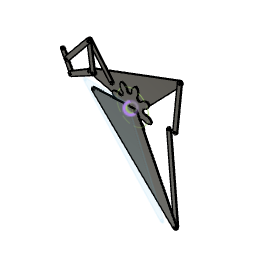
CAD (Autodesk Fusion 360 design; units mm, degrees)
description: Spur Gear; Module: 2.0; Num Teeth: 8; Pressure Angle: 20.0; Backlash: 0.00 mm
Autodesk Fusion 360 part; units mm, degrees
note: some values were not read from the file. Set by a fixed rule: which sketch regions a step uses.
(part 1 of 2)
sketch "Sketch2" plane through (0, 0, 0) normal (0, 1, 0) x (1, 0, 0)
  line L0 (20.2187, -3.6863) -> (18.4977, -4.9158)
  arc A0 (18.4977, -4.9158) -> (19.6603, -6.5431) centre (19.079, -5.7294) ccw
  line L1 (19.6603, -6.5431) -> (21.3813, -5.3137)
  arc A1 (21.3813, -5.3137) -> (20.2187, -3.6863) centre (20.8, -4.5) ccw
  line L2 (20.8, -4.5) -> (19.079, -5.7294) construction
  line L3 (19.079, -5.7294) -> (20.8, -4.5)
  circle A2 centre (19.079, -5.7294) radius 0.5
  circle A3 centre (20.8, -4.5) radius 0.5
  dimension "d10" = 2
  dimension "d11" = 1
  dimension "d12" = 1
  constraint tangent L0 A0
  constraint tangent A0 L1
  constraint parallel L0 L1
  constraint tangent L1 A1
  constraint tangent L0 A1
  constraint coincident A0.centre L2.end
  constraint coincident A1.centre L2.start
  constraint concentric A0 A2
  constraint concentric A1 A3
  measures "d10" diameter of A0
  measures "d11" diameter of A2
  measures "d12" diameter of A3
sketch "Sketch3" plane through (0, 0, 0) normal (0, 1, 0) x (1, 0, 0)
  line L0 (40.363, -4.4753) -> (54.2331, 34.1031)
  arc A0 (54.2331, 34.1031) -> (52.351, 34.7797) centre (53.2921, 34.4414) ccw
  line L1 (52.351, 34.7797) -> (38.481, -3.7987)
  arc A1 (38.481, -3.7987) -> (40.363, -4.4753) centre (39.422, -4.137) ccw
  line L2 (39.422, -4.137) -> (53.2921, 34.4414) construction
  line L3 (39.422, -4.137) -> (53.2921, 34.4414)
  circle A2 centre (39.422, -4.137) radius 0.5
  circle A3 centre (53.2921, 34.4414) radius 0.5
  dimension "d17" = 2
  dimension "d18" = 1
  dimension "d19" = 1
  constraint tangent L0 A0
  constraint tangent A0 L1
  constraint parallel L0 L1
  constraint tangent L1 A1
  constraint tangent L0 A1
  constraint coincident A1.centre L2.start
  constraint coincident A0.centre L2.end
  constraint concentric A1 A2
  constraint concentric A0 A3
  measures "d17" diameter of A0
  measures "d18" diameter of A2
  measures "d19" diameter of A3
extrude "Extrude2" add sketch "Sketch3" against normal blind 0.5 makes body 1
sketch "Sketch4" plane through (0, 0, 0) normal (0, 1, 0) x (1, 0, 0)
  line L0 (41.629, -4.9251) -> (52.2449, -24.6941)
  arc A0 (52.2449, -24.6941) -> (54.0069, -23.7479) centre (53.1259, -24.221) ccw
  line L1 (54.0069, -23.7479) -> (43.391, -3.9789)
  arc A1 (43.391, -3.9789) -> (41.629, -4.9251) centre (42.51, -4.452) ccw
  line L2 (42.51, -4.452) -> (53.1259, -24.221) construction
  line L3 (42.51, -4.452) -> (53.1259, -24.221)
  circle A2 centre (42.51, -4.452) radius 0.5
  circle A3 centre (53.1259, -24.221) radius 0.5
  dimension "d24" = 2
  dimension "d25" = 1
  dimension "d26" = 1
  constraint tangent L0 A0
  constraint tangent A0 L1
  constraint parallel L0 L1
  constraint tangent L1 A1
  constraint tangent L0 A1
  constraint coincident A1.centre L2.start
  constraint coincident A0.centre L2.end
  constraint concentric A1 A2
  constraint concentric A0 A3
  measures "d24" diameter of A0
  measures "d25" diameter of A2
  measures "d26" diameter of A3
extrude "Extrude3" add sketch "Sketch4" against normal blind 0.5 separate body makes body 2
sketch "Sketch5" plane through (0, 0, 0) normal (0, 1, 0) x (1, 0, 0)
  line L0 (-13.1989, -13.1062) -> (-9.6831, -4.2011)
  arc A0 (-9.6831, -4.2011) -> (-11.5434, -3.4667) centre (-10.6133, -3.8339) ccw
  line L1 (-11.5434, -3.4667) -> (-15.0591, -12.3718)
  arc A1 (-15.0591, -12.3718) -> (-13.1989, -13.1062) centre (-14.129, -12.739) ccw
  line L2 (-14.129, -12.739) -> (-10.6133, -3.8339) construction
  line L3 (-14.129, -12.739) -> (-10.6133, -3.8339)
  circle A2 centre (-14.129, -12.739) radius 0.5
  circle A3 centre (-10.6133, -3.8339) radius 0.5
  dimension "d32" = 2
  dimension "d33" = 1
  dimension "d34" = 1
  constraint tangent L0 A0
  constraint tangent A0 L1
  constraint parallel L0 L1
  constraint tangent L1 A1
  constraint tangent L0 A1
  constraint coincident A1.centre L2.start
  constraint coincident A0.centre L2.end
  constraint concentric A1 A2
  constraint concentric A0 A3
  measures "d32" diameter of A0
  measures "d33" diameter of A2
  measures "d34" diameter of A3
extrude "Extrude4" add sketch "Sketch5" against normal blind 0.5 separate body makes body 3
copy_body "Body->Comp1" bodies 2 removing the originals makes body 4 in component "Component"
copy_body "Body->Comp2" bodies 1 removing the originals makes body 5 in component "Component'"
copy_body "Body->Comp4" bodies 3 removing the originals makes body 6 in component "Component''"
sketch "Sketch8" plane through (0, 0, 0) normal (0, 1, 0) x (1, 0, 0)
  line L0 (-5, -5) -> (5, -5)
  line L1 (5, -5) -> (5, 2.5)
  line L2 (5, 2.5) -> (-5, 2.5)
  line L3 (-5, 2.5) -> (-5, -5)
  constraint horizontal L0
  constraint vertical L1
  constraint horizontal L2
  constraint vertical L3
extrude "Extrude5" add sketch "Sketch8" along normal blind 0.5 separate body makes body 7
copy_body "Body->Comp5" bodies 7 removing the originals makes body 8 in component "Component'''"
sketch "Sketch9" plane through (0, 0, 0) normal (0, 1, 0) x (1, 0, 0)
  line L0 (-1, -1) -> (1, -1)
  line L1 (1, -1) -> (1, 1)
  line L2 (1, 1) -> (-1, 1)
  line L3 (-1, 1) -> (-1, -1)
  constraint horizontal L0
  constraint vertical L1
  constraint horizontal L2
  constraint vertical L3
extrude "Extrude6" add sketch "Sketch9" along normal blind 0.5 separate body makes body 9
copy_body "Body->Comp6" bodies 9 removing the originals makes body 10 in component "Component''''"
sketch "Sketch10" plane through (0, 0, 0) normal (0, 1, 0) x (1, 0, 0)
  line L0 (-1, -1) -> (1, -1)
  line L1 (1, -1) -> (1, 1)
  line L2 (1, 1) -> (-1, 1)
  line L3 (-1, 1) -> (-1, -1)
  constraint horizontal L0
  constraint vertical L1
  constraint horizontal L2
  constraint vertical L3
extrude "Extrude7" add sketch "Sketch10" along normal blind 0.5 separate body makes body 11
copy_body "Body->Comp7" bodies 11 removing the originals makes body 12 in component "Component'''''"
sketch "Sketch11" plane through (0, 0, 0) normal (0, 1, 0) x (1, 0, 0)
  line L0 (-0.5, -0.5) -> (0.5, -0.5)
  line L1 (0.5, -0.5) -> (0.5, 0.5)
  line L2 (0.5, 0.5) -> (-0.5, 0.5)
  line L3 (-0.5, 0.5) -> (-0.5, -0.5)
  constraint horizontal L0
  constraint vertical L1
  constraint horizontal L2
  constraint vertical L3
extrude "Extrude8" add sketch "Sketch11" along normal blind 0.5 separate body makes body 13
copy_body "Body->Comp8" bodies 13 removing the originals makes body 14 in component "Component''''''"
sketch "Sketch14" plane through (0, 0, 0) normal (0, 1, 0) x (1, 0, 0)
  line L0 (0, 0) -> (4.9713, -9.3835)
  line L1 (4.9713, -9.3835) -> (6.8938, -11.5466)
  line L2 (6.8938, -11.5466) -> (0, 0)
  line L3 (-19.2227, 34.1473) -> (4.144, -9.9579)
  line L4 (4.144, -9.9579) -> (13.1804, -20.1253)
  line L5 (13.1804, -20.1253) -> (-19.2227, 34.1473)
  circle A0 centre (0, 0) radius 1
  circle A1 centre (6.8938, -11.5466) radius 1
  circle A2 centre (4.9713, -9.3835) radius 1
  circle A3 centre (6.8938, -11.5466) radius 0.5
  circle A4 centre (4.9713, -9.3835) radius 0.5
  circle A5 centre (0, 0) radius 0.5
  dimension "d87" = 10.619
  dimension "d88" = 2.894
  dimension "d89" = 13.448
  dimension "d90" = 1
  dimension "d91" = 1
  dimension "d92" = 1
  dimension "d93" = 1
  constraint coincident L0.start L2.end
  constraint coincident L1.end L2.start
  constraint tangent L4 A1
  constraint coincident L0.end L1.start
  constraint tangent L3 A2
  constraint concentric A1 A3
  constraint concentric A2 A4
  measures "d87" distance of L0.start L0.end
  measures "d88" distance of L0.end L1.end
  measures "d89" distance of L1.end L0.start
  measures "d91" diameter of A3
  measures "d92" diameter of A4
  measures "d93" diameter of A5
extrude "Extrude10" add sketch "Sketch14" against normal blind 0.5 separate body contours L0 L2 A0 A5 | L0 L2 A0 A5 | L0 L2 A0 A2 | L0 L3 A0 A2 | L2 L5 A0 A1 A2 | L0 L1 L2 A2 A4 | L0 L1 A2 A4 | L2 A2 | L1 L2 A1 A2 | L1 L4 A1 A2 | L1 L2 A1 A3 | L1 L2 A1 A3 makes body 15
copy_body "Body->Comp9" bodies 15 removing the originals makes body 16 in component "Component'''''''"
sketch "Sketch15" plane through (0, 0, 0) normal (0, 1, 0) x (1, 0, 0)
  line L0 (-1, 0) -> (-1, -13.5)
  arc A0 (-1, -13.5) -> (1, -13.5) centre (0, -13.5) ccw
  line L1 (1, -13.5) -> (1, 0)
  arc A1 (1, 0) -> (-1, 0) centre (0, 0) ccw
  line L2 (0, 0) -> (0, -13.5) construction
  circle A2 centre (0, -13.5) radius 0.5
  circle A3 centre (0, 0) radius 0.5
  dimension "d100" = 2
  dimension "d101" = 1
  dimension "d102" = 1
  constraint tangent L0 A0
  constraint tangent A0 L1
  constraint parallel L0 L1
  constraint tangent L1 A1
  constraint tangent L0 A1
  constraint vertical L2
  constraint coincident A1.centre L2.start
  constraint concentric A0 A2
  constraint concentric A1 A3
  measures "d100" diameter of A0
  measures "d101" diameter of A2
  measures "d102" diameter of A3
extrude "Extrude11" add sketch "Sketch15" against normal blind 0.5 separate body makes body 17
copy_body "Body->Comp10" bodies 17 removing the originals makes body 18 in component "Component''''''''"
sketch "Sketch16" plane through (0, 0, 0) normal (0, 1, 0) x (1, 0, 0)
  line L0 (-2, -2) -> (2, -2)
  line L1 (2, -2) -> (2, 30)
  line L2 (2, 30) -> (-2, 30)
  line L3 (-2, 30) -> (-2, -2)
  constraint horizontal L0
  constraint vertical L1
  constraint horizontal L2
  constraint vertical L3
extrude "Extrude12" add sketch "Sketch16" along normal blind 0.5 separate body makes body 19
copy_body "Body->Comp11" bodies 19 removing the originals makes body 20 in component "Component'''''''''"
sketch "Sketch17" plane through (0, 0, 0) normal (0, 1, 0) x (1, 0, 0)
  line L0 (5.9221, 49.648) -> (29.8072, 28.8562)
  line L1 (5.9221, 49.648) -> (-16.9692, 41.844)
  line L2 (-16.9692, 41.844) -> (29.8072, 28.8562)
  line L3 (6.1444, 50.7803) -> (33.7942, 26.7114)
  line L4 (-20.355, 41.7463) -> (33.7942, 26.7114)
  line L5 (6.1444, 50.7803) -> (-20.355, 41.7463)
  circle A0 centre (29.8072, 28.8562) radius 1
  circle A1 centre (-16.9692, 41.844) radius 1
  circle A2 centre (5.9221, 49.648) radius 1
  circle A3 centre (5.9221, 49.648) radius 0.5
  circle A4 centre (29.8072, 28.8562) radius 0.5
  circle A5 centre (-16.9692, 41.844) radius 0.5
  dimension "d111" = 50
  dimension "d112" = 31.667
  dimension "d113" = 24.185
  dimension "d114" = 48.546
  dimension "d115" = 1
  dimension "d116" = 1
  dimension "d117" = 1
  dimension "d118" = 1
  constraint coincident L0.end L2.end
  constraint tangent L4 A0
  constraint coincident L1.end L2.start
  constraint tangent L4 A1
  constraint coincident L0.start L1.start
  constraint tangent L3 A2
  constraint concentric A2 A3
  constraint concentric A0 A4
  constraint concentric A1 A5
  measures "d111" distance of origin L0.start
  measures "d112" distance of L0.start L0.end
  measures "d113" distance of L0.start L1.end
  measures "d114" distance of L1.end L0.end
  measures "d116" diameter of A3
  measures "d117" diameter of A4
  measures "d118" diameter of A5
extrude "Extrude13" add sketch "Sketch17" against normal blind 0.5 separate body contours L0 L1 A2 A3 | L0 L1 A2 A3 | L0 L3 A0 A2 | L0 L1 L2 A0 A1 A2 | L1 L5 A1 A2 | L0 L2 A0 A4 | L0 L2 A0 A4 | L1 L2 A1 A5 | L1 L2 A1 A5 | L2 L4 A0 A1 makes body 21
copy_body "Body->Comp12" bodies 21 removing the originals makes body 22 in component "Component''''''''''"
sketch "Sketch18" plane through (0, 0, 0) normal (0, 1, 0) x (1, 0, 0)
  line L0 (0, 40) -> (28.0014, 75.7058)
  line L1 (0, 40) -> (-20.2217, 44.9555)
  line L2 (-20.2217, 44.9555) -> (28.0014, 75.7058)
  line L3 (0.3887, 38.8752) -> (32.4039, 79.6992)
  line L4 (-22.7316, 44.541) -> (32.4039, 79.6992)
  line L5 (0.3887, 38.8752) -> (-22.7316, 44.541)
  circle A0 centre (0, 40) radius 1
  circle A1 centre (-20.2217, 44.9555) radius 1
  circle A2 centre (28.0014, 75.7058) radius 1
  circle A3 centre (-20.2217, 44.9555) radius 0.5
  circle A4 centre (0, 40) radius 0.5
  circle A5 centre (28.0014, 75.7058) radius 0.5
  dimension "d129" = 40
  dimension "d130" = 45.376
  dimension "d131" = 20.82
  dimension "d132" = 57.193
  dimension "d133" = 1
  dimension "d134" = 1
  dimension "d135" = 1
  dimension "d136" = 1
  constraint coincident L0.end L2.end
  constraint coincident L0.start L1.start
  constraint tangent L5 A0
  constraint coincident L1.end L2.start
  constraint tangent L5 A1
  constraint tangent L3 A2
  constraint concentric A1 A3
  constraint concentric A0 A4
  constraint concentric A2 A5
  measures "d129" distance of origin L0.start
  measures "d130" distance of L0.start L0.end
  measures "d131" distance of L0.start L1.end
  measures "d132" distance of L1.end L0.end
  measures "d134" diameter of A3
  measures "d135" diameter of A4
  measures "d136" diameter of A5
extrude "Extrude14" add sketch "Sketch18" against normal blind 0.5 separate body contours L0 L1 A0 A4 | L0 L1 A0 A4 | L0 L1 L2 A0 A1 A2 | L0 L3 A0 A2 | L1 L5 A0 A1 | L0 L2 A2 A5 | L0 L2 A2 A5 | L1 L2 A1 A3 | L1 L2 A1 A3 | L2 L4 A1 A2 makes body 23
copy_body "Body->Comp13" bodies 23 removing the originals makes body 24 in component "Component'''''''''''"
sketch "Sketch19" plane through (0, 0, 0) normal (0, 1, 0) x (1, 0, 0)
  circle A0 centre (0, 20) radius 1
  circle A1 centre (0, 20) radius 0.5
  dimension "d151" = 20
  dimension "d152" = 2
  dimension "d153" = 1
  constraint concentric A0 A1
  measures "d151" distance of origin A0.centre
  measures "d152" diameter of A0
  measures "d153" diameter of A1
extrude "Extrude15" add sketch "Sketch19" along normal blind 0.5 separate body makes body 25
chamfer "Chamfer1" distance 0.1 angle 45 1 edges at (-0.9323, 0, -19.6384) on bodies 25
chamfer "Chamfer2" distance 0.1 angle 45 1 edges at (-0.9323, 0.5, -19.6384) on bodies 25
chamfer "Chamfer3" distance 0.1 angle 45 2 edges at (-0.4662, 0, -20.1808) (-0.4662, 0.5, -20.1808) on bodies 25
copy_body "Body->Comp14" bodies 25 removing the originals makes body 26 in component "Component''''''''''''"
move_face "OffsetFaces1" offset -16 1 faces at (-0.6667, 0.1667, 2) on bodies 20 in component "Component'''''''''"
sketch "Sketch20" plane through (0, 0, 0) normal (0, 1, 0) x (1, 0, 0)
  line L0 (-10, 0) -> (-14, 0)
  line L1 (-14, 0) -> (-14, 16)
  line L2 (-10, 0) -> (-10, 16)
  line L3 (-10, 16) -> (-14, 16)
  dimension "d168" = 10
  dimension "d169" = 4
  dimension "d170" = 16
  dimension "d171" = 16
  constraint perpendicular L0 L1
  constraint perpendicular L1 L3
  measures "d168" distance of origin L0.start
  measures "d169" distance of L0.start L0.end
  measures "d170" distance of L0.end L1.end
  measures "d171" distance of L0.start L2.end
extrude "Extrude16" add sketch "Sketch20" along normal blind 0.5 separate body makes body 27
copy_body "Body->Comp15" bodies 27 removing the originals makes body 28 in component "Component'''''''''''''"
sketch "Sketch21" plane through (0, 0, 0) normal (0, 1, 0) x (1, 0, 0)
  line L0 (-39, 0) -> (-39, 17)
  arc A0 (-39, 17) -> (-41, 17) centre (-40, 17) ccw
  line L1 (-41, 17) -> (-41, 0)
  arc A1 (-41, 0) -> (-39, 0) centre (-40, 0) ccw
  line L2 (-40, 0) -> (-40, 17) construction
  circle A2 centre (-40, 0) radius 0.5
  circle A3 centre (-40, 17) radius 0.5
  dimension "d182" = 40
  dimension "d183" = 2
  dimension "d184" = 1
  dimension "d185" = 1
  constraint tangent L0 A0
  constraint tangent A0 L1
  constraint parallel L0 L1
  constraint tangent L1 A1
  constraint tangent L0 A1
  constraint concentric A1 A2
  constraint concentric A0 A3
  measures "d182" distance of origin A1.centre
  measures "d183" diameter of A0
  measures "d184" diameter of A2
  measures "d185" diameter of A3
extrude "Extrude17" add sketch "Sketch21" along normal blind 0.5 separate body makes body 29
copy_body "Body->Comp16" bodies 29 removing the originals makes body 30 in component "Component''''''''''''''"
sketch "Sketch22" plane through (0, 0, 0) normal (0, 1, 0) x (1, 0, 0)
  line L0 (-24, 0) -> (-24, 17)
  arc A0 (-24, 17) -> (-26, 17) centre (-25, 17) ccw
  line L1 (-26, 17) -> (-26, 0)
  arc A1 (-26, 0) -> (-24, 0) centre (-25, 0) ccw
  line L2 (-25, 0) -> (-25, 17) construction
  circle A2 centre (-25, 0) radius 0.5
  circle A3 centre (-25, 17) radius 0.5
  dimension "d189" = 25
  dimension "d190" = 2
  dimension "d191" = 1
  dimension "d192" = 1
  constraint tangent L0 A0
  constraint tangent A0 L1
  constraint parallel L0 L1
  constraint tangent L1 A1
  constraint tangent L0 A1
  constraint concentric A1 A2
  constraint concentric A0 A3
  measures "d189" distance of origin A1.centre
  measures "d190" diameter of A0
  measures "d191" diameter of A2
  measures "d192" diameter of A3
extrude "Extrude18" add sketch "Sketch22" along normal blind 0.5 separate body makes body 31
copy_body "Body->Comp17" bodies 31 removing the originals makes body 32 in component "Component'''''''''''''''"
sketch "Sketch23" plane through (0, 0, 0) normal (0, 1, 0) x (1, 0, 0)
  line L0 (-20, 0) -> (-16, 0)
  line L1 (-20, 0) -> (-20, 16)
  line L2 (-16, 0) -> (-16, 16)
  line L3 (-20, 16) -> (-16, 16)
  line L4 (-14.5, 0) -> (-10.5, 0)
  line L5 (-14.5, 0) -> (-14.5, 16)
  line L6 (-10.5, 0) -> (-10.5, 16)
  line L7 (-14.5, 16) -> (-10.5, 16)
  line L8 (-20, 17) -> (-16, 17)
  line L9 (-16, 17) -> (-16, 33)
  line L10 (-20, 17) -> (-20, 33)
  line L11 (-20, 33) -> (-16, 33)
  line L12 (-10, 17) -> (-14, 17)
  line L13 (-14, 17) -> (-14, 33)
  line L14 (-10, 17) -> (-10, 33)
  line L15 (-14, 33) -> (-10, 33)
  dimension "d195" = 4
  dimension "d196" = 16
  dimension "d197" = 16
  dimension "d198" = 4
  dimension "d199" = 16
  dimension "d200" = 16
  dimension "d201" = 16
  dimension "d202" = 16
  dimension "d203" = 4
  dimension "d204" = 16
  dimension "d205" = 16
  constraint perpendicular L0 L1
  constraint perpendicular L0 L2
  constraint perpendicular L4 L5
  constraint perpendicular L4 L6
  constraint horizontal L8
  constraint perpendicular L8 L9
  constraint perpendicular L8 L10
  constraint perpendicular L9 L12
  constraint perpendicular L12 L13
  constraint perpendicular L12 L14
  measures "d195" distance of L0.start L0.end
  measures "d196" distance of L0.start L1.end
  measures "d197" distance of L0.end L2.end
  measures "d198" distance of L4.start L4.end
  measures "d199" distance of L4.start L5.end
  measures "d200" distance of L4.end L6.end
  measures "d201" distance of L8.end L9.end
  measures "d202" distance of L8.start L10.end
  measures "d203" distance of L12.start L12.end
  measures "d204" distance of L12.end L13.end
  measures "d205" distance of L12.start L14.end
extrude "Extrude19" add sketch "Sketch23" along normal blind 0.5 separate body makes body 33 at (-11.8333, 0, -5.3333) makes body 34 at (-18.6667, 0, -22.3333) makes body 35 at (-18.6667, 0, -10.6667) makes body 36 at (-11.3333, 0, -22.3333)
copy_body "Body->Comp18" bodies 35 removing the originals makes body 37 in component "Component''''''''''''''''"
copy_body "Body->Comp19" bodies 33 removing the originals makes body 38 in component "Component'''''''''''''''''"
copy_body "Body->Comp20" bodies 34 removing the originals makes body 39 in component "Component''''''''''''''''''"
copy_body "Body->Comp21" bodies 36 removing the originals makes body 40 in component "Component'''''''''''''''''''"
sketch "Sketch24" plane through (0, 0, 0) normal (0, 1, 0) x (1, 0, 0)
  line L0 (0, 0) -> (0, -14.2)
  line L1 (0, -14.2) -> (3.4641, -12.2)
  line L2 (0, -14.2) -> (4, -14.2) construction
  line L3 (0, -14.2) -> (-3.4641, -12.2)
  dimension "d216" = 14.2
  dimension "d217" = 30
  dimension "d218" = 4
  constraint coincident L0.start origin
  constraint vertical L0
  constraint horizontal L2
  constraint symmetric L1.start L0 L2.start
  constraint symmetric L0 L1.end L3.end
  measures "d216" distance of L0.start L0.end
  measures "d217" angle of L1 L2
  measures "d218" distance of L0.end L1.end
sketch "Sketch1" plane through (0, 0, 0) normal (0, 0, 1) x (1, 0, 0) in component "Spur Gear (8 teeth)"
  circle A0 centre (0, 0) radius 5.5492
  circle A1 centre (0, 0) radius 0.5
extrude "Extrude1" add sketch "Sketch1" along normal blind 0.5 separate body makes body 41 in component "Spur Gear (8 teeth)"
sketch "Sketch2 (2)" plane through (0, 0, 0) normal (0, 0, 1) x (1, 0, 0) in component "Spur Gear (8 teeth)"
  spline S0 degree 5 poles (7.3504, -1.5763) (7.3577, -1.5779) (7.3723, -1.5807) (7.3943, -1.5841) (7.4239, -1.5871) (7.4612, -1.5888) (7.4987, -1.5889) (7.5364, -1.588) (7.5741, -1.5866) (7.6119, -1.5849) (7.6498, -1.5827) (7.6877, -1.5801) (7.7257, -1.5767) (7.7638, -1.5726) (7.802, -1.5677) (7.8402, -1.562) (7.8785, -1.5558) (7.9168, -1.549) (7.9551, -1.5418) (7.9935, -1.5341) (8.0319, -1.526) (8.0703, -1.5174) (8.1087, -1.5082) (8.1471, -1.4986) (8.1856, -1.4885) (8.224, -1.4779) (8.2624, -1.4668) (8.3009, -1.4553) (8.3393, -1.4434) (8.3778, -1.4311) (8.4162, -1.4183) (8.4546, -1.4051) (8.4929, -1.3915) (8.5313, -1.3774) (8.5696, -1.363) (8.608, -1.3481) (8.6462, -1.3328) (8.6845, -1.3172) (8.7227, -1.3011) (8.7609, -1.2847) (8.799, -1.2679) (8.8371, -1.2506) (8.8752, -1.2331) (8.9132, -1.2151) (8.9512, -1.1967) (8.9891, -1.178) (9.0269, -1.1589) (9.0647, -1.1395) (9.1025, -1.1197) (9.1401, -1.0995) (9.1778, -1.079) (9.2153, -1.0581) (9.2528, -1.0368) (9.2902, -1.0152) (9.3276, -0.9933) (9.3648, -0.971) (9.402, -0.9484) (9.4392, -0.9254) (9.4762, -0.9021) (9.5132, -0.8784) (9.55, -0.8544) (9.5868, -0.8301) (9.6235, -0.8055) (9.6602, -0.7805) (9.6967, -0.7552) (9.7331, -0.7295) (9.7695, -0.7036) (9.8057, -0.6773) (9.8418, -0.6507) (9.8779, -0.6238) (9.9138, -0.5965) (9.9425, -0.5745) (9.9639, -0.5578) (9.9782, -0.5466) (9.9854, -0.541) knots 0 0 0 0 0 0 0.01428571 0.02857143 0.04285714 0.05714286 0.07142857 0.08571429 0.1 0.11428571 0.12857143 0.14285714 0.15714286 0.17142857 0.18571429 0.2 0.21428571 0.22857143 0.24285714 0.25714286 0.27142857 0.28571429 0.3 0.31428571 0.32857143 0.34285714 0.35714286 0.37142857 0.38571429 0.4 0.41428571 0.42857143 0.44285714 0.45714286 0.47142857 0.48571429 0.5 0.51428571 0.52857143 0.54285714 0.55714286 0.57142857 0.58571429 0.6 0.61428571 0.62857143 0.64285714 0.65714286 0.67142857 0.68571429 0.7 0.71428571 0.72857143 0.74285714 0.75714286 0.77142857 0.78571429 0.8 0.81428571 0.82857143 0.84285714 0.85714286 0.87142857 0.88571429 0.9 0.91428571 0.92857143 0.94285714 0.95714286 0.97142857 0.98571429 1 1 1 1 1 1
  spline S1 degree 5 poles (7.3504, 1.5763) (7.3577, 1.5779) (7.3723, 1.5807) (7.3943, 1.5841) (7.4239, 1.5871) (7.4612, 1.5888) (7.4987, 1.5889) (7.5364, 1.588) (7.5741, 1.5866) (7.6119, 1.5849) (7.6498, 1.5827) (7.6877, 1.5801) (7.7257, 1.5767) (7.7638, 1.5726) (7.802, 1.5677) (7.8402, 1.562) (7.8785, 1.5558) (7.9168, 1.549) (7.9551, 1.5418) (7.9935, 1.5341) (8.0319, 1.526) (8.0703, 1.5174) (8.1087, 1.5082) (8.1471, 1.4986) (8.1856, 1.4885) (8.224, 1.4779) (8.2624, 1.4668) (8.3009, 1.4553) (8.3393, 1.4434) (8.3778, 1.4311) (8.4162, 1.4183) (8.4546, 1.4051) (8.4929, 1.3915) (8.5313, 1.3774) (8.5696, 1.363) (8.608, 1.3481) (8.6462, 1.3328) (8.6845, 1.3172) (8.7227, 1.3011) (8.7609, 1.2847) (8.799, 1.2679) (8.8371, 1.2506) (8.8752, 1.2331) (8.9132, 1.2151) (8.9512, 1.1967) (8.9891, 1.178) (9.0269, 1.1589) (9.0647, 1.1395) (9.1025, 1.1197) (9.1401, 1.0995) (9.1778, 1.079) (9.2153, 1.0581) (9.2528, 1.0368) (9.2902, 1.0152) (9.3276, 0.9933) (9.3648, 0.971) (9.402, 0.9484) (9.4392, 0.9254) (9.4762, 0.9021) (9.5132, 0.8784) (9.55, 0.8544) (9.5868, 0.8301) (9.6235, 0.8055) (9.6602, 0.7805) (9.6967, 0.7552) (9.7331, 0.7295) (9.7695, 0.7036) (9.8057, 0.6773) (9.8418, 0.6507) (9.8779, 0.6238) (9.9138, 0.5965) (9.9425, 0.5745) (9.9639, 0.5578) (9.9782, 0.5466) (9.9854, 0.541) knots 0 0 0 0 0 0 0.01428571 0.02857143 0.04285714 0.05714286 0.07142857 0.08571429 0.1 0.11428571 0.12857143 0.14285714 0.15714286 0.17142857 0.18571429 0.2 0.21428571 0.22857143 0.24285714 0.25714286 0.27142857 0.28571429 0.3 0.31428571 0.32857143 0.34285714 0.35714286 0.37142857 0.38571429 0.4 0.41428571 0.42857143 0.44285714 0.45714286 0.47142857 0.48571429 0.5 0.51428571 0.52857143 0.54285714 0.55714286 0.57142857 0.58571429 0.6 0.61428571 0.62857143 0.64285714 0.65714286 0.67142857 0.68571429 0.7 0.71428571 0.72857143 0.74285714 0.75714286 0.77142857 0.78571429 0.8 0.81428571 0.82857143 0.84285714 0.85714286 0.87142857 0.88571429 0.9 0.91428571 0.92857143 0.94285714 0.95714286 0.97142857 0.98571429 1 1 1 1 1 1
  arc A0 (9.9854, -0.541) -> (9.9854, 0.541) centre (0, 0) ccw
  line L0 (5.4161, -1.1636) -> (7.3504, -1.5763)
  line L1 (5.4161, 1.1636) -> (7.3504, 1.5763)
  line L2 (5.4161, -1.1636) -> (5.4161, 1.1636)
  point P0 (7.5292, -1.5881)
  point P1 (7.7124, -1.5778)
  point P2 (7.8984, -1.5522)
  point P3 (8.0864, -1.5135)
  point P4 (8.2759, -1.4628)
  point P5 (8.4663, -1.4008)
  point P6 (8.6575, -1.3282)
  point P7 (8.8489, -1.2451)
  point P8 (9.0403, -1.152)
  point P9 (9.2313, -1.049)
  point P10 (9.4216, -0.9362)
  point P11 (9.611, -0.8139)
  point P12 (9.799, -0.6821)
  point P13 (7.5292, 1.5881)
  point P14 (7.7124, 1.5778)
  point P15 (7.8984, 1.5522)
  point P16 (8.0864, 1.5135)
  point P17 (8.2759, 1.4628)
  point P18 (8.4663, 1.4008)
  point P19 (8.6575, 1.3282)
  point P20 (8.8489, 1.2451)
  point P21 (9.0403, 1.152)
  point P22 (9.2313, 1.049)
  point P23 (9.4216, 0.9362)
  point P24 (9.611, 0.8139)
  point P25 (9.799, 0.6821)
extrude "Extrude2'" add sketch "Sketch2 (2)" along normal blind 0.5 bodies 41 in component "Spur Gear (8 teeth)"
fillet "Fillet1" radius 1 2 edges at (5.4254, -1.1656, 0.25) (5.4254, 1.1656, 0.25) on bodies 41 in component "Spur Gear (8 teeth)"
pattern_circular "C-Pattern1" count 8 over 360 about axis through (0, 0, 0) along (0, 0, 1) of "Extrude2'", "Fillet1" in component "Spur Gear (8 teeth)"
sketch "Sketch3 (2)" plane through (0, 0, 0) normal (0, 0, 1) x (1, 0, 0) in component "Spur Gear (8 teeth)"
  circle A0 centre (0, 0) radius 8 construction
sketch "Sketch26" plane through (0, -1, 0) normal (0, -1, 0) x (1, 0, 0)
  circle A0 centre (36.5077, -36.7553) radius 0.5
  circle A1 centre (-2.0699, 5.468) radius 0.5
  circle A2 centre (18.7448, 4.9995) radius 0.5
  arc A3 (19.665, 5.391) -> (18.7673, 5.9992) centre (18.7448, 4.9995) ccw
  line L0 (18.7673, 5.9992) -> (-2.0474, 6.4678)
  arc A4 (-2.0474, 6.4678) -> (-2.8081, 4.7935) centre (-2.0699, 5.468) ccw
  line L1 (-2.8081, 4.7935) -> (35.7694, -37.4298)
  arc A5 (35.7694, -37.4298) -> (37.4279, -36.3638) centre (36.5077, -36.7553) ccw
  line L2 (37.4279, -36.3638) -> (19.665, 5.391)
  point P0 (20.8, 4.5)
sketch "Sketch27" plane through (0, -0.25, 0) normal (0, -1, 0) x (1, 0, 0)
  arc A0 (56.2039, -3.3739) -> (56.3228, -3.0869) centre (51.1385, -1.1076) ccw
  arc A1 (57.4657, -2.4656) -> (56.3228, -3.0869) centre (57.257, -3.4436) ccw
  line L0 (57.4657, -2.4656) -> (58.489, -2.684)
  spline S0 degree 5 poles (58.489, -2.684) (58.4963, -2.6855) (58.5109, -2.6883) (58.5329, -2.6918) (58.5625, -2.6948) (58.5998, -2.6964) (58.6373, -2.6965) (58.6749, -2.6956) (58.7127, -2.6943) (58.7505, -2.6925) (58.7883, -2.6904) (58.8263, -2.6877) (58.8643, -2.6844) (58.9024, -2.6802) (58.9405, -2.6753) (58.9788, -2.6697) (59.017, -2.6634) (59.0554, -2.6566) (59.0937, -2.6494) (59.1321, -2.6417) (59.1704, -2.6336) (59.2088, -2.625) (59.2472, -2.6159) (59.2857, -2.6063) (59.3241, -2.5961) (59.3625, -2.5855) (59.401, -2.5745) (59.4394, -2.563) (59.4779, -2.551) (59.5163, -2.5387) (59.5547, -2.5259) (59.5931, -2.5127) (59.6315, -2.4991) (59.6699, -2.4851) (59.7082, -2.4706) (59.7465, -2.4558) (59.7848, -2.4405) (59.823, -2.4248) (59.8613, -2.4088) (59.8994, -2.3923) (59.9376, -2.3755) (59.9757, -2.3583) (60.0137, -2.3407) (60.0517, -2.3227) (60.0897, -2.3044) (60.1276, -2.2857) (60.1655, -2.2666) (60.2033, -2.2471) (60.241, -2.2273) (60.2787, -2.2071) (60.3163, -2.1866) (60.3539, -2.1657) (60.3914, -2.1445) (60.4288, -2.1229) (60.4661, -2.1009) (60.5034, -2.0786) (60.5406, -2.056) (60.5777, -2.033) (60.6148, -2.0097) (60.6517, -1.9861) (60.6886, -1.9621) (60.7254, -1.9378) (60.7621, -1.9131) (60.7987, -1.8881) (60.8352, -1.8628) (60.8717, -1.8372) (60.908, -1.8112) (60.9442, -1.7849) (60.9804, -1.7583) (61.0164, -1.7314) (61.0524, -1.7041) (61.081, -1.6821) (61.1025, -1.6654) (61.1168, -1.6542) (61.1239, -1.6486) knots 0 0 0 0 0 0 0.01428571 0.02857143 0.04285714 0.05714286 0.07142857 0.08571429 0.1 0.11428571 0.12857143 0.14285714 0.15714286 0.17142857 0.18571429 0.2 0.21428571 0.22857143 0.24285714 0.25714286 0.27142857 0.28571429 0.3 0.31428571 0.32857143 0.34285714 0.35714286 0.37142857 0.38571429 0.4 0.41428571 0.42857143 0.44285714 0.45714286 0.47142857 0.48571429 0.5 0.51428571 0.52857143 0.54285714 0.55714286 0.57142857 0.58571429 0.6 0.61428571 0.62857143 0.64285714 0.65714286 0.67142857 0.68571429 0.7 0.71428571 0.72857143 0.74285714 0.75714286 0.77142857 0.78571429 0.8 0.81428571 0.82857143 0.84285714 0.85714286 0.87142857 0.88571429 0.9 0.91428571 0.92857143 0.94285714 0.95714286 0.97142857 0.98571429 1 1 1 1 1 1
  arc A2 (61.1239, -1.6486) -> (61.1239, -0.5666) centre (51.1385, -1.1076) ccw
  spline S1 degree 5 poles (61.1239, -0.5666) (61.1168, -0.561) (61.1025, -0.5499) (61.081, -0.5332) (61.0524, -0.5111) (61.0164, -0.4839) (60.9804, -0.457) (60.9442, -0.4304) (60.908, -0.4041) (60.8717, -0.3781) (60.8352, -0.3525) (60.7987, -0.3272) (60.7621, -0.3022) (60.7254, -0.2775) (60.6886, -0.2532) (60.6517, -0.2292) (60.6148, -0.2055) (60.5777, -0.1822) (60.5406, -0.1593) (60.5034, -0.1366) (60.4661, -0.1143) (60.4288, -0.0924) (60.3914, -0.0708) (60.3539, -0.0496) (60.3163, -0.0287) (60.2787, -0.0081) (60.241, 0.012) (60.2033, 0.0318) (60.1655, 0.0513) (60.1276, 0.0704) (60.0897, 0.0891) (60.0517, 0.1075) (60.0137, 0.1254) (59.9757, 0.143) (59.9376, 0.1602) (59.8994, 0.1771) (59.8613, 0.1935) (59.823, 0.2095) (59.7848, 0.2252) (59.7465, 0.2405) (59.7082, 0.2553) (59.6699, 0.2698) (59.6315, 0.2838) (59.5931, 0.2975) (59.5547, 0.3106) (59.5163, 0.3234) (59.4779, 0.3358) (59.4394, 0.3477) (59.401, 0.3592) (59.3625, 0.3703) (59.3241, 0.3809) (59.2857, 0.391) (59.2472, 0.4006) (59.2088, 0.4097) (59.1704, 0.4183) (59.1321, 0.4265) (59.0937, 0.4341) (59.0554, 0.4414) (59.017, 0.4481) (58.9788, 0.4544) (58.9405, 0.46) (58.9024, 0.4649) (58.8643, 0.4691) (58.8263, 0.4724) (58.7883, 0.4751) (58.7505, 0.4772) (58.7127, 0.479) (58.6749, 0.4804) (58.6373, 0.4812) (58.5998, 0.4811) (58.5625, 0.4795) (58.5329, 0.4765) (58.5109, 0.4731) (58.4963, 0.4702) (58.489, 0.4687) knots -1 -1 -1 -1 -1 -1 -0.98571429 -0.97142857 -0.95714286 -0.94285714 -0.92857143 -0.91428571 -0.9 -0.88571429 -0.87142857 -0.85714286 -0.84285714 -0.82857143 -0.81428571 -0.8 -0.78571429 -0.77142857 -0.75714286 -0.74285714 -0.72857143 -0.71428571 -0.7 -0.68571429 -0.67142857 -0.65714286 -0.64285714 -0.62857143 -0.61428571 -0.6 -0.58571429 -0.57142857 -0.55714286 -0.54285714 -0.52857143 -0.51428571 -0.5 -0.48571429 -0.47142857 -0.45714286 -0.44285714 -0.42857143 -0.41428571 -0.4 -0.38571429 -0.37142857 -0.35714286 -0.34285714 -0.32857143 -0.31428571 -0.3 -0.28571429 -0.27142857 -0.25714286 -0.24285714 -0.22857143 -0.21428571 -0.2 -0.18571429 -0.17142857 -0.15714286 -0.14285714 -0.12857143 -0.11428571 -0.1 -0.08571429 -0.07142857 -0.05714286 -0.04285714 -0.02857143 -0.01428571 0 0 0 0 0 0
  line L1 (58.489, 0.4687) -> (57.4657, 0.2503)
  arc A3 (56.3228, 0.8717) -> (57.4657, 0.2503) centre (57.257, 1.2283) ccw
  arc A4 (56.3228, 0.8717) -> (56.2039, 1.1586) centre (51.1385, -1.1076) ccw
  arc A5 (56.5727, 2.4061) -> (56.2039, 1.1586) centre (57.1167, 1.567) ccw
  line L2 (56.5727, 2.4061) -> (57.4507, 2.9753)
  spline S2 degree 5 poles (57.4507, 2.9753) (57.457, 2.9793) (57.4693, 2.9876) (57.4873, 3.0008) (57.5103, 3.0196) (57.5378, 3.0448) (57.5644, 3.0713) (57.5905, 3.0985) (57.6162, 3.1262) (57.6417, 3.1541) (57.6669, 3.1824) (57.6919, 3.2111) (57.7164, 3.2404) (57.7404, 3.2702) (57.7639, 3.3007) (57.7869, 3.3317) (57.8096, 3.3632) (57.8319, 3.3951) (57.8539, 3.4273) (57.8756, 3.4599) (57.897, 3.4927) (57.918, 3.526) (57.9387, 3.5596) (57.9591, 3.5936) (57.9791, 3.6279) (57.9988, 3.6626) (58.0182, 3.6976) (58.0372, 3.7329) (58.056, 3.7685) (58.0744, 3.8044) (58.0926, 3.8406) (58.1104, 3.8771) (58.1279, 3.9139) (58.1451, 3.9509) (58.162, 3.9882) (58.1786, 4.0258) (58.1948, 4.0637) (58.2108, 4.1018) (58.2265, 4.1402) (58.2418, 4.1788) (58.2569, 4.2177) (58.2717, 4.2568) (58.2862, 4.2962) (58.3003, 4.3357) (58.3142, 4.3756) (58.3278, 4.4156) (58.341, 4.4559) (58.354, 4.4964) (58.3667, 4.5371) (58.3791, 4.578) (58.3911, 4.6191) (58.4029, 4.6604) (58.4144, 4.7019) (58.4256, 4.7437) (58.4365, 4.7856) (58.4471, 4.8277) (58.4574, 4.87) (58.4674, 4.9125) (58.4771, 4.9552) (58.4865, 4.998) (58.4956, 5.0411) (58.5045, 5.0843) (58.513, 5.1277) (58.5212, 5.1712) (58.5291, 5.215) (58.5368, 5.2589) (58.5441, 5.3029) (58.5511, 5.3471) (58.5579, 5.3915) (58.5643, 5.436) (58.5705, 5.4807) (58.5751, 5.5166) (58.5785, 5.5435) (58.5807, 5.5615) (58.5818, 5.5705) knots 0 0 0 0 0 0 0.01428571 0.02857143 0.04285714 0.05714286 0.07142857 0.08571429 0.1 0.11428571 0.12857143 0.14285714 0.15714286 0.17142857 0.18571429 0.2 0.21428571 0.22857143 0.24285714 0.25714286 0.27142857 0.28571429 0.3 0.31428571 0.32857143 0.34285714 0.35714286 0.37142857 0.38571429 0.4 0.41428571 0.42857143 0.44285714 0.45714286 0.47142857 0.48571429 0.5 0.51428571 0.52857143 0.54285714 0.55714286 0.57142857 0.58571429 0.6 0.61428571 0.62857143 0.64285714 0.65714286 0.67142857 0.68571429 0.7 0.71428571 0.72857143 0.74285714 0.75714286 0.77142857 0.78571429 0.8 0.81428571 0.82857143 0.84285714 0.85714286 0.87142857 0.88571429 0.9 0.91428571 0.92857143 0.94285714 0.95714286 0.97142857 0.98571429 1 1 1 1 1 1
  arc A6 (58.5818, 5.5705) -> (57.8167, 6.3356) centre (51.1385, -1.1076) ccw
  spline S3 degree 5 poles (57.8167, 6.3356) (57.8077, 6.3345) (57.7897, 6.3323) (57.7627, 6.329) (57.7269, 6.3243) (57.6822, 6.3181) (57.6377, 6.3117) (57.5933, 6.3049) (57.5491, 6.2979) (57.505, 6.2906) (57.4612, 6.2829) (57.4174, 6.275) (57.3739, 6.2668) (57.3305, 6.2583) (57.2873, 6.2494) (57.2442, 6.2403) (57.2014, 6.2309) (57.1587, 6.2212) (57.1162, 6.2112) (57.0739, 6.2009) (57.0318, 6.1903) (56.9898, 6.1794) (56.9481, 6.1682) (56.9066, 6.1567) (56.8653, 6.145) (56.8241, 6.1329) (56.7832, 6.1205) (56.7425, 6.1078) (56.7021, 6.0949) (56.6618, 6.0816) (56.6217, 6.068) (56.5819, 6.0541) (56.5424, 6.04) (56.503, 6.0255) (56.4639, 6.0107) (56.425, 5.9957) (56.3864, 5.9803) (56.348, 5.9646) (56.3099, 5.9486) (56.272, 5.9324) (56.2344, 5.9158) (56.1971, 5.8989) (56.16, 5.8817) (56.1233, 5.8642) (56.0868, 5.8464) (56.0506, 5.8282) (56.0147, 5.8098) (55.9791, 5.7911) (55.9438, 5.772) (55.9088, 5.7526) (55.8741, 5.733) (55.8397, 5.7129) (55.8058, 5.6926) (55.7722, 5.6718) (55.7389, 5.6508) (55.706, 5.6294) (55.6735, 5.6077) (55.6413, 5.5857) (55.6094, 5.5634) (55.5779, 5.5408) (55.5469, 5.5177) (55.5164, 5.4942) (55.4866, 5.4702) (55.4573, 5.4457) (55.4286, 5.4208) (55.4003, 5.3955) (55.3723, 5.37) (55.3447, 5.3443) (55.3174, 5.3182) (55.291, 5.2917) (55.2658, 5.2642) (55.247, 5.2411) (55.2338, 5.2231) (55.2255, 5.2108) (55.2214, 5.2045) knots -1 -1 -1 -1 -1 -1 -0.98571429 -0.97142857 -0.95714286 -0.94285714 -0.92857143 -0.91428571 -0.9 -0.88571429 -0.87142857 -0.85714286 -0.84285714 -0.82857143 -0.81428571 -0.8 -0.78571429 -0.77142857 -0.75714286 -0.74285714 -0.72857143 -0.71428571 -0.7 -0.68571429 -0.67142857 -0.65714286 -0.64285714 -0.62857143 -0.61428571 -0.6 -0.58571429 -0.57142857 -0.55714286 -0.54285714 -0.52857143 -0.51428571 -0.5 -0.48571429 -0.47142857 -0.45714286 -0.44285714 -0.42857143 -0.41428571 -0.4 -0.38571429 -0.37142857 -0.35714286 -0.34285714 -0.32857143 -0.31428571 -0.3 -0.28571429 -0.27142857 -0.25714286 -0.24285714 -0.22857143 -0.21428571 -0.2 -0.18571429 -0.17142857 -0.15714286 -0.14285714 -0.12857143 -0.11428571 -0.1 -0.08571429 -0.07142857 -0.05714286 -0.04285714 -0.02857143 -0.01428571 0 0 0 0 0 0
  line L3 (55.2214, 5.2045) -> (54.6523, 4.3265)
  arc A7 (53.4048, 3.9577) -> (54.6523, 4.3265) centre (53.8132, 4.8705) ccw
  arc A8 (53.4048, 3.9577) -> (53.1178, 4.0766) centre (51.1385, -1.1076) ccw
  arc A9 (52.4965, 5.2195) -> (53.1178, 4.0766) centre (53.4745, 5.0108) ccw
  line L4 (52.4965, 5.2195) -> (52.7149, 6.2428)
  spline S4 degree 5 poles (52.7149, 6.2428) (52.7164, 6.2501) (52.7193, 6.2647) (52.7227, 6.2867) (52.7257, 6.3163) (52.7273, 6.3536) (52.7274, 6.3911) (52.7266, 6.4287) (52.7252, 6.4665) (52.7234, 6.5043) (52.7213, 6.5422) (52.7186, 6.5801) (52.7153, 6.6181) (52.7111, 6.6562) (52.7062, 6.6944) (52.7006, 6.7326) (52.6943, 6.7709) (52.6875, 6.8092) (52.6803, 6.8475) (52.6726, 6.8859) (52.6645, 6.9242) (52.6559, 6.9626) (52.6468, 7.0011) (52.6372, 7.0395) (52.6271, 7.0779) (52.6165, 7.1164) (52.6054, 7.1548) (52.5939, 7.1933) (52.582, 7.2317) (52.5696, 7.2701) (52.5568, 7.3085) (52.5436, 7.3469) (52.53, 7.3853) (52.516, 7.4237) (52.5015, 7.462) (52.4867, 7.5003) (52.4714, 7.5386) (52.4557, 7.5769) (52.4397, 7.6151) (52.4232, 7.6533) (52.4064, 7.6914) (52.3892, 7.7295) (52.3716, 7.7675) (52.3536, 7.8056) (52.3353, 7.8435) (52.3166, 7.8814) (52.2975, 7.9193) (52.278, 7.9571) (52.2582, 7.9948) (52.238, 8.0325) (52.2175, 8.0701) (52.1966, 8.1077) (52.1754, 8.1452) (52.1538, 8.1826) (52.1318, 8.2199) (52.1096, 8.2572) (52.0869, 8.2944) (52.064, 8.3315) (52.0406, 8.3686) (52.017, 8.4055) (51.993, 8.4424) (51.9687, 8.4792) (51.944, 8.5159) (51.919, 8.5525) (51.8937, 8.5891) (51.8681, 8.6255) (51.8421, 8.6618) (51.8158, 8.6981) (51.7892, 8.7342) (51.7623, 8.7702) (51.7351, 8.8062) (51.713, 8.8348) (51.6963, 8.8563) (51.6852, 8.8706) (51.6795, 8.8777) knots 0 0 0 0 0 0 0.01428571 0.02857143 0.04285714 0.05714286 0.07142857 0.08571429 0.1 0.11428571 0.12857143 0.14285714 0.15714286 0.17142857 0.18571429 0.2 0.21428571 0.22857143 0.24285714 0.25714286 0.27142857 0.28571429 0.3 0.31428571 0.32857143 0.34285714 0.35714286 0.37142857 0.38571429 0.4 0.41428571 0.42857143 0.44285714 0.45714286 0.47142857 0.48571429 0.5 0.51428571 0.52857143 0.54285714 0.55714286 0.57142857 0.58571429 0.6 0.61428571 0.62857143 0.64285714 0.65714286 0.67142857 0.68571429 0.7 0.71428571 0.72857143 0.74285714 0.75714286 0.77142857 0.78571429 0.8 0.81428571 0.82857143 0.84285714 0.85714286 0.87142857 0.88571429 0.9 0.91428571 0.92857143 0.94285714 0.95714286 0.97142857 0.98571429 1 1 1 1 1 1
  arc A10 (51.6795, 8.8777) -> (50.5976, 8.8777) centre (51.1385, -1.1076) ccw
  spline S5 degree 5 poles (50.5976, 8.8777) (50.5919, 8.8706) (50.5808, 8.8563) (50.5641, 8.8348) (50.542, 8.8062) (50.5148, 8.7702) (50.4879, 8.7342) (50.4613, 8.6981) (50.435, 8.6618) (50.409, 8.6255) (50.3834, 8.5891) (50.3581, 8.5525) (50.3331, 8.5159) (50.3084, 8.4792) (50.2841, 8.4424) (50.2601, 8.4055) (50.2365, 8.3686) (50.2131, 8.3315) (50.1902, 8.2944) (50.1675, 8.2572) (50.1453, 8.2199) (50.1233, 8.1826) (50.1017, 8.1452) (50.0805, 8.1077) (50.0596, 8.0701) (50.0391, 8.0325) (50.0189, 7.9948) (49.9991, 7.9571) (49.9796, 7.9193) (49.9605, 7.8814) (49.9418, 7.8435) (49.9235, 7.8056) (49.9055, 7.7675) (49.8879, 7.7295) (49.8707, 7.6914) (49.8539, 7.6533) (49.8374, 7.6151) (49.8214, 7.5769) (49.8057, 7.5386) (49.7904, 7.5003) (49.7756, 7.462) (49.7611, 7.4237) (49.7471, 7.3853) (49.7335, 7.3469) (49.7203, 7.3085) (49.7075, 7.2701) (49.6951, 7.2317) (49.6832, 7.1933) (49.6717, 7.1548) (49.6606, 7.1164) (49.65, 7.0779) (49.6399, 7.0395) (49.6303, 7.0011) (49.6212, 6.9626) (49.6126, 6.9242) (49.6045, 6.8859) (49.5968, 6.8475) (49.5895, 6.8092) (49.5828, 6.7709) (49.5765, 6.7326) (49.5709, 6.6944) (49.566, 6.6562) (49.5618, 6.6181) (49.5585, 6.5801) (49.5558, 6.5422) (49.5537, 6.5043) (49.5519, 6.4665) (49.5505, 6.4287) (49.5497, 6.3911) (49.5498, 6.3536) (49.5514, 6.3163) (49.5544, 6.2867) (49.5578, 6.2647) (49.5607, 6.2501) (49.5622, 6.2428) knots -1 -1 -1 -1 -1 -1 -0.98571429 -0.97142857 -0.95714286 -0.94285714 -0.92857143 -0.91428571 -0.9 -0.88571429 -0.87142857 -0.85714286 -0.84285714 -0.82857143 -0.81428571 -0.8 -0.78571429 -0.77142857 -0.75714286 -0.74285714 -0.72857143 -0.71428571 -0.7 -0.68571429 -0.67142857 -0.65714286 -0.64285714 -0.62857143 -0.61428571 -0.6 -0.58571429 -0.57142857 -0.55714286 -0.54285714 -0.52857143 -0.51428571 -0.5 -0.48571429 -0.47142857 -0.45714286 -0.44285714 -0.42857143 -0.41428571 -0.4 -0.38571429 -0.37142857 -0.35714286 -0.34285714 -0.32857143 -0.31428571 -0.3 -0.28571429 -0.27142857 -0.25714286 -0.24285714 -0.22857143 -0.21428571 -0.2 -0.18571429 -0.17142857 -0.15714286 -0.14285714 -0.12857143 -0.11428571 -0.1 -0.08571429 -0.07142857 -0.05714286 -0.04285714 -0.02857143 -0.01428571 0 0 0 0 0 0
  line L5 (49.5622, 6.2428) -> (49.7806, 5.2195)
  arc A11 (49.1593, 4.0766) -> (49.7806, 5.2195) centre (48.8026, 5.0108) ccw
  arc A12 (49.1593, 4.0766) -> (48.8723, 3.9577) centre (51.1385, -1.1076) ccw
  arc A13 (47.6248, 4.3265) -> (48.8723, 3.9577) centre (48.4639, 4.8705) ccw
  line L6 (47.6248, 4.3265) -> (47.0556, 5.2045)
  spline S6 degree 5 poles (47.0556, 5.2045) (47.0516, 5.2108) (47.0433, 5.2231) (47.0301, 5.2411) (47.0113, 5.2642) (46.9861, 5.2917) (46.9597, 5.3182) (46.9324, 5.3443) (46.9048, 5.37) (46.8768, 5.3955) (46.8485, 5.4208) (46.8198, 5.4457) (46.7905, 5.4702) (46.7607, 5.4942) (46.7302, 5.5177) (46.6992, 5.5408) (46.6677, 5.5634) (46.6358, 5.5857) (46.6036, 5.6077) (46.5711, 5.6294) (46.5382, 5.6508) (46.5049, 5.6718) (46.4713, 5.6926) (46.4374, 5.7129) (46.403, 5.733) (46.3683, 5.7526) (46.3333, 5.772) (46.298, 5.7911) (46.2624, 5.8098) (46.2265, 5.8282) (46.1903, 5.8464) (46.1538, 5.8642) (46.117, 5.8817) (46.08, 5.8989) (46.0427, 5.9158) (46.0051, 5.9324) (45.9672, 5.9486) (45.9291, 5.9646) (45.8907, 5.9803) (45.8521, 5.9957) (45.8132, 6.0107) (45.7741, 6.0255) (45.7347, 6.04) (45.6952, 6.0541) (45.6554, 6.068) (45.6153, 6.0816) (45.575, 6.0949) (45.5346, 6.1078) (45.4939, 6.1205) (45.453, 6.1329) (45.4118, 6.145) (45.3705, 6.1567) (45.329, 6.1682) (45.2873, 6.1794) (45.2453, 6.1903) (45.2032, 6.2009) (45.1609, 6.2112) (45.1184, 6.2212) (45.0757, 6.2309) (45.0329, 6.2403) (44.9898, 6.2494) (44.9466, 6.2583) (44.9032, 6.2668) (44.8597, 6.275) (44.8159, 6.2829) (44.7721, 6.2906) (44.728, 6.2979) (44.6838, 6.3049) (44.6394, 6.3117) (44.5949, 6.3181) (44.5502, 6.3243) (44.5144, 6.329) (44.4874, 6.3323) (44.4694, 6.3345) (44.4604, 6.3356) knots 0 0 0 0 0 0 0.01428571 0.02857143 0.04285714 0.05714286 0.07142857 0.08571429 0.1 0.11428571 0.12857143 0.14285714 0.15714286 0.17142857 0.18571429 0.2 0.21428571 0.22857143 0.24285714 0.25714286 0.27142857 0.28571429 0.3 0.31428571 0.32857143 0.34285714 0.35714286 0.37142857 0.38571429 0.4 0.41428571 0.42857143 0.44285714 0.45714286 0.47142857 0.48571429 0.5 0.51428571 0.52857143 0.54285714 0.55714286 0.57142857 0.58571429 0.6 0.61428571 0.62857143 0.64285714 0.65714286 0.67142857 0.68571429 0.7 0.71428571 0.72857143 0.74285714 0.75714286 0.77142857 0.78571429 0.8 0.81428571 0.82857143 0.84285714 0.85714286 0.87142857 0.88571429 0.9 0.91428571 0.92857143 0.94285714 0.95714286 0.97142857 0.98571429 1 1 1 1 1 1
  arc A14 (44.4604, 6.3356) -> (43.6953, 5.5705) centre (51.1385, -1.1076) ccw
  spline S7 degree 5 poles (43.6953, 5.5705) (43.6964, 5.5615) (43.6986, 5.5435) (43.702, 5.5166) (43.7066, 5.4807) (43.7128, 5.436) (43.7192, 5.3915) (43.726, 5.3471) (43.733, 5.3029) (43.7403, 5.2589) (43.748, 5.215) (43.7559, 5.1712) (43.7641, 5.1277) (43.7726, 5.0843) (43.7815, 5.0411) (43.7906, 4.998) (43.8, 4.9552) (43.8097, 4.9125) (43.8197, 4.87) (43.83, 4.8277) (43.8406, 4.7856) (43.8515, 4.7437) (43.8627, 4.7019) (43.8742, 4.6604) (43.886, 4.6191) (43.898, 4.578) (43.9104, 4.5371) (43.9231, 4.4964) (43.9361, 4.4559) (43.9493, 4.4156) (43.9629, 4.3756) (43.9768, 4.3357) (43.9909, 4.2962) (44.0054, 4.2568) (44.0202, 4.2177) (44.0353, 4.1788) (44.0506, 4.1402) (44.0663, 4.1018) (44.0823, 4.0637) (44.0985, 4.0258) (44.1151, 3.9882) (44.132, 3.9509) (44.1492, 3.9139) (44.1667, 3.8771) (44.1845, 3.8406) (44.2027, 3.8044) (44.2211, 3.7685) (44.2399, 3.7329) (44.2589, 3.6976) (44.2783, 3.6626) (44.298, 3.6279) (44.318, 3.5936) (44.3384, 3.5596) (44.3591, 3.526) (44.3801, 3.4927) (44.4015, 3.4599) (44.4232, 3.4273) (44.4452, 3.3951) (44.4675, 3.3632) (44.4902, 3.3317) (44.5132, 3.3007) (44.5367, 3.2702) (44.5607, 3.2404) (44.5852, 3.2111) (44.6102, 3.1824) (44.6354, 3.1541) (44.6609, 3.1262) (44.6866, 3.0985) (44.7127, 3.0713) (44.7393, 3.0448) (44.7668, 3.0196) (44.7898, 3.0008) (44.8078, 2.9876) (44.8201, 2.9793) (44.8264, 2.9753) knots -1 -1 -1 -1 -1 -1 -0.98571429 -0.97142857 -0.95714286 -0.94285714 -0.92857143 -0.91428571 -0.9 -0.88571429 -0.87142857 -0.85714286 -0.84285714 -0.82857143 -0.81428571 -0.8 -0.78571429 -0.77142857 -0.75714286 -0.74285714 -0.72857143 -0.71428571 -0.7 -0.68571429 -0.67142857 -0.65714286 -0.64285714 -0.62857143 -0.61428571 -0.6 -0.58571429 -0.57142857 -0.55714286 -0.54285714 -0.52857143 -0.51428571 -0.5 -0.48571429 -0.47142857 -0.45714286 -0.44285714 -0.42857143 -0.41428571 -0.4 -0.38571429 -0.37142857 -0.35714286 -0.34285714 -0.32857143 -0.31428571 -0.3 -0.28571429 -0.27142857 -0.25714286 -0.24285714 -0.22857143 -0.21428571 -0.2 -0.18571429 -0.17142857 -0.15714286 -0.14285714 -0.12857143 -0.11428571 -0.1 -0.08571429 -0.07142857 -0.05714286 -0.04285714 -0.02857143 -0.01428571 0 0 0 0 0 0
  line L7 (44.8264, 2.9753) -> (45.7044, 2.4061)
  arc A15 (46.0732, 1.1586) -> (45.7044, 2.4061) centre (45.1604, 1.567) ccw
  arc A16 (46.0732, 1.1586) -> (45.9543, 0.8717) centre (51.1385, -1.1076) ccw
  arc A17 (44.8114, 0.2503) -> (45.9543, 0.8717) centre (45.0201, 1.2283) ccw
  line L8 (44.8114, 0.2503) -> (43.7881, 0.4687)
  spline S8 degree 5 poles (43.7881, 0.4687) (43.7808, 0.4702) (43.7662, 0.4731) (43.7442, 0.4765) (43.7146, 0.4795) (43.6773, 0.4811) (43.6398, 0.4812) (43.6022, 0.4804) (43.5644, 0.479) (43.5266, 0.4772) (43.4888, 0.4751) (43.4508, 0.4724) (43.4128, 0.4691) (43.3747, 0.4649) (43.3366, 0.46) (43.2983, 0.4544) (43.2601, 0.4481) (43.2217, 0.4414) (43.1834, 0.4341) (43.145, 0.4265) (43.1067, 0.4183) (43.0683, 0.4097) (43.0299, 0.4006) (42.9914, 0.391) (42.953, 0.3809) (42.9145, 0.3703) (42.8761, 0.3592) (42.8377, 0.3477) (42.7992, 0.3358) (42.7608, 0.3234) (42.7224, 0.3106) (42.684, 0.2975) (42.6456, 0.2838) (42.6072, 0.2698) (42.5689, 0.2553) (42.5306, 0.2405) (42.4923, 0.2252) (42.4541, 0.2095) (42.4158, 0.1935) (42.3777, 0.1771) (42.3395, 0.1602) (42.3014, 0.143) (42.2634, 0.1254) (42.2254, 0.1075) (42.1874, 0.0891) (42.1495, 0.0704) (42.1116, 0.0513) (42.0738, 0.0318) (42.0361, 0.012) (41.9984, -0.0081) (41.9608, -0.0287) (41.9232, -0.0496) (41.8857, -0.0708) (41.8483, -0.0924) (41.811, -0.1143) (41.7737, -0.1366) (41.7365, -0.1593) (41.6994, -0.1822) (41.6623, -0.2055) (41.6254, -0.2292) (41.5885, -0.2532) (41.5517, -0.2775) (41.515, -0.3022) (41.4784, -0.3272) (41.4419, -0.3525) (41.4054, -0.3781) (41.3691, -0.4041) (41.3329, -0.4304) (41.2967, -0.457) (41.2607, -0.4839) (41.2247, -0.5111) (41.1961, -0.5332) (41.1746, -0.5499) (41.1603, -0.561) (41.1532, -0.5666) knots 0 0 0 0 0 0 0.01428571 0.02857143 0.04285714 0.05714286 0.07142857 0.08571429 0.1 0.11428571 0.12857143 0.14285714 0.15714286 0.17142857 0.18571429 0.2 0.21428571 0.22857143 0.24285714 0.25714286 0.27142857 0.28571429 0.3 0.31428571 0.32857143 0.34285714 0.35714286 0.37142857 0.38571429 0.4 0.41428571 0.42857143 0.44285714 0.45714286 0.47142857 0.48571429 0.5 0.51428571 0.52857143 0.54285714 0.55714286 0.57142857 0.58571429 0.6 0.61428571 0.62857143 0.64285714 0.65714286 0.67142857 0.68571429 0.7 0.71428571 0.72857143 0.74285714 0.75714286 0.77142857 0.78571429 0.8 0.81428571 0.82857143 0.84285714 0.85714286 0.87142857 0.88571429 0.9 0.91428571 0.92857143 0.94285714 0.95714286 0.97142857 0.98571429 1 1 1 1 1 1
  arc A18 (41.1532, -0.5666) -> (41.1532, -1.6486) centre (51.1385, -1.1076) ccw